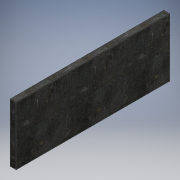
# Autodesk Inventor part: 内层正板
Saved by Autodesk Inventor 2017 (Build 210142000, 142)
## iProperties
Part Number: 内层正板
Material: 常规
Document SubType Name: Modeling
Designer: PANDA
Density: 1 g/cm^3
Appearance: 默认
Author: PANDA
Autodesk Inventor part; units mm, degrees
ref_plane "YZ Plane" through (0, 0, 0) normal (1, 0, 0) x (0, 1, 0)
ref_plane "XZ Plane" through (0, 0, 0) normal (0, 1, 0) x (-1, 0, 0)
ref_plane "XY Plane" through (0, 0, 0) normal (0, 0, 1) x (1, 0, 0)
sketch "草图1" plane through (0, 0, 0) normal (1, 0, 0) x (0, 1, 0)
  line L0 (230, 90) -> (-230, 90)
  line L1 (-230, 90) -> (-230, -90)
  line L2 (-230, -90) -> (230, -90)
  line L3 (230, -90) -> (230, 90)
  point P0 (0, 0)
  dimension "d0" = 460
  dimension "d1" = 180
  constraints: 8 end point, 2 parallel, 1 horizontal, 1 perpendicular
  measures "d0" distance of L2.end L1.end
  measures "d1" distance of L1.end L0.end
extrude "拉伸1" add sketch "草图1" along normal blind 20
sketch "草图2" plane through (0, -230, -90) normal (0, -1, 0) x (1, 0, 0)
  circle A0 centre (10, 30) radius 2
  point P0 (0, 90)
  dimension "d4" = 4
  constraints: 1 centre point
  measures "d4" diameter of A0
extrude "拉伸2" cut sketch "草图2" against normal blind 40
sketch "草图3" plane through (0, -230, -90) normal (0, -1, 0) x (1, 0, 0)
  circle A0 centre (10, 150) radius 2
  point P0 (0, 90)
  dimension "d7" = 4
  constraints: 1 centre point
  measures "d7" diameter of A0
extrude "拉伸3" cut sketch "草图3" against normal blind 40
sketch "草图4" plane through (0, 230, 90) normal (0, 1, 0) x (1, 0, 0)
  line L0 (20, 0) -> (20, 180) projected
  line L1 (0, 0) -> (20, 0)
  line L2 (20, 0) -> (20, 180)
  line L3 (20, 180) -> (0, 180)
  line L4 (0, 180) -> (0, 0)
  point P0 (0, 90)
  constraints: 8 end point, 2 parallel, 1 horizontal, 1 perpendicular
extrude "拉伸4" cut sketch "草图4" against normal blind 60
sketch "草图5" plane through (0, 170, 90) normal (0, 1, 0) x (1, 0, 0)
  line L0 (0, 0) -> (0, 180) projected
  line L1 (0, 0) -> (20, 0) projected
  line L2 (0, 180) -> (20, 180)
  line L3 (20, 180) -> (20, 0)
  line L4 (20, 0) -> (0, 0)
  line L5 (0, 0) -> (0, 180)
  point P0 (0, 90)
  constraints: 8 end point, 2 parallel, 1 horizontal, 1 perpendicular
extrude "拉伸5" add sketch "草图5" along normal blind 50
sketch "草图6" plane through (0, 0, 0) normal (-1, 0, 0) x (0, 0, 1)
  circle A0 centre (0, 200) radius 5
  point P0 (0, 0)
  dimension "d14" = 10
  constraints: 1 centre point
  measures "d14" diameter of A0
extrude "拉伸6" cut sketch "草图6" against normal through all
sketch "草图7" plane through (0, 220, 90) normal (0, 1, 0) x (1, 0, 0)
  line L0 (0, 0) -> (20, 0) projected
  line L1 (20, 0) -> (0, 0)
  line L2 (0, 0) -> (0, 180)
  line L3 (0, 180) -> (20, 180)
  line L4 (20, 180) -> (20, 0)
  point P0 (0, 90)
  constraints: 8 end point, 2 parallel, 1 horizontal, 1 perpendicular
extrude "拉伸7" add sketch "草图7" along normal blind 20
fillet "圆角1" radius 2 2 edges at (8, -190, 60) (8, -190, -60)
fillet "圆角1" radius 2 16 edges at (10, 240, 90) (0, 5, 90) (10, -230, 90) (20, 5, 90) (20, 240, 0) (20, -230, 0) (20, 5, -90) (20, 200, -5) (0, 240, 0) (0, 5, -90) (0, -230, 0) (0, 200, -5) (10, 240, -90) (10, -230, -90) (8, -230, 60) (8, -230, -60)
